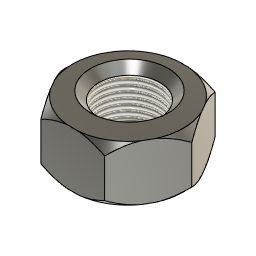
Day #6 - Hex Nut v2 (Autodesk Fusion 360 design; units mm, degrees)
Autodesk Fusion 360 part; units mm, degrees
sketch "Hex Polygon" plane through (0, 0, 0) normal (0, 0, 1) x (1, 0, 0) in component "Hex Nut"
  line L0 (-5.7735, 10) -> (-11.547, 0)
  line L1 (-11.547, 0) -> (-5.7735, -10)
  line L2 (-5.7735, -10) -> (5.7735, -10)
  line L3 (5.7735, -10) -> (11.547, 0)
  line L4 (11.547, 0) -> (5.7735, 10)
  line L5 (5.7735, 10) -> (-5.7735, 10)
  dimension "d1" = 10
  constraint horizontal L5
  measures "d1" distance of origin L5
extrude "Extrude1" add sketch "Hex Polygon" along normal blind 10 in component "Hex Nut"
sketch "Chamfer Cutout" plane through (0, 0, 0) normal (0, 1, 0) x (1, 0, 0) in component "Hex Nut"
  line L0 (11.547, -10) -> (10.047, -10)
  line L1 (10.047, -10) -> (11.547, -8.5)
  line L2 (11.547, -8.5) -> (11.547, -10)
  point P0 (11.547, -10)
  dimension "d4" = 1.5
  constraint coincident P0 L0.start
  constraint horizontal L0
  constraint perpendicular L0 L2
  constraint equal L0 L2
  measures "d4" distance of P0 L1.end
revolve "Revolve1" cut sketch "Chamfer Cutout" angle 360 about axis through (0, 0, 1.75) along (0, 0, 1) in component "Hex Nut"
hole "Hole1" at (-0.7219, 0.9887, 10) direction (0, 0, -1) diameter 11.035 end through all countersink diameter 14 countersink angle 90 in component "Hex Nut"
thread "Thread1" "GB Metric profile 12.0 M12x1 6H" thread offset 0 thread depth 8.5 in component "Hex Nut"
ref_plane "WorkPlane1" through (0, 0, 5) normal (0, 0, 1) x (1, 0, 0) in component "Hex Nut"
mirror "Mirror1" about plane through (0, 0, 5) normal (0, 0, 1) of 7 faces at (10.7886, 0.4867, 9.2475) (4.9728, -9.5865, 9.2475) (-4.9728, -9.5865, 9.2475) (0.1071, -8.6444, 10) (4.9728, 9.5865, 9.2475) (-10.7886, -0.4867, 9.2475) (-4.9728, 9.5865, 9.2475) in component "Hex Nut"
component "Hex Nut" placed x (1, 0, 0) y (0, 1, 0) z (0, 0, 1) at (0, 0, 0)
named bodies: "Hex Nut"
